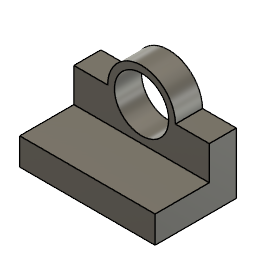
Exercise_3 Problem (Autodesk Fusion 360 design; units mm, degrees)
part number: 2026-05-18-23-03-23-890
Autodesk Fusion 360 part; units mm, degrees
note: some values were not read from the file. Set by a fixed rule: which sketch regions a step uses.
sketch "Sketch1" plane through (0, 0, 0) normal (0, 1, 0) x (1, 0, 0)
  line L0 (50, 30) -> (25, 30)
  line L1 (-50, 10) -> (-50, -30)
  line L2 (-50, -30) -> (50, -30)
  line L3 (50, -30) -> (50, 10)
  line L4 (50, 30) -> (-50, -30) construction
  line L5 (-50, 30) -> (50, -30) construction
  line L6 (-50, 30) -> (-50, 10)
  line L7 (-50, 10) -> (50, 10)
  line L8 (50, 10) -> (50, 30)
  line L9 (-50, 30) -> (0, 30)
  arc A0 (25, 30) -> (-25, 30) centre (0, 30) ccw
  line L10 (0, 30) -> (25, 30)
  circle A1 centre (0, 30) radius 20
  dimension "d1" = 100
  dimension "d2" = 60
  dimension "d3" = 20
  dimension "d4" = 50
  dimension "d5" = 40
  constraint horizontal L0
  constraint perpendicular L0 L1
  constraint parallel L0 L2
  constraint parallel L1 L3
  constraint coincident L4 origin
  constraint coincident L5 origin
  constraint perpendicular L0 L6
  constraint perpendicular L3 L7
  constraint coincident L9.end A0.centre
  constraint coincident L0 L9.end
  constraint concentric A0 A1
  measures "d1" distance of L1.end L2.end
  measures "d2" distance of L5.start L1.end
  measures "d3" distance of L5.start L1.start
  measures "d4" diameter of A0
  measures "d5" diameter of A1
extrude "Extrude1" add sketch "Sketch1" along normal blind 20 contours L1 L2 L3 L7
extrude "Extrude2" add sketch "Sketch1" along normal blind 45 contours L0 L7 L8 L10 A1 | L6 L7 L9 A1 | L9 L10 A1 picked at (-13.2655, 29.0512)
sketch "Sketch2" plane through (0, 0, -10) normal (0, 0, 1) x (1, 0, 0)
  line L0 (-50, 20) -> (50, 20)
  line L1 (50, 20) -> (50, 45)
  line L2 (50, 45) -> (-50, 45)
  line L3 (-50, 45) -> (-50, 20)
  line L4 (-50, 45) -> (0, 45)
  circle A0 centre (0, 45) radius 20
  arc A1 (25, 45) -> (-25, 45) centre (0, 45) ccw
  dimension "d10" = 50
  dimension "d11" = 40
  constraint coincident L2.end L3.start
  constraint midpoint L2 L4.end
  constraint coincident L4.end A0.centre
  constraint concentric A0 A1
  constraint coincident L2 A1.end
  constraint coincident L2 A1.start
  measures "d10" diameter of A1
  measures "d11" diameter of A0
extrude "Extrude3" add sketch "Sketch2" against normal blind 20 contours L2 L4 A0 A1
extrude "Extrude4" cut sketch "Sketch2" against normal blind 20 contours L2 L4 A0 picked at (13.2589, 44.0064)
